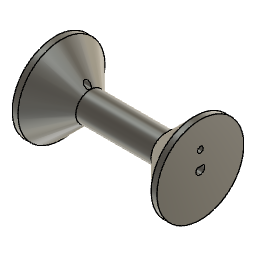
rouleau v1 (Autodesk Fusion 360 design; units mm, degrees)
Autodesk Fusion 360 part; units mm, degrees
sketch "Esquisse1" plane through (0, 0, 0) normal (0, 1, 0) x (1, 0, 0)
  line L0 (-25, -1.5) -> (-25, -15)
  line L1 (-25, -15) -> (-23, -15)
  line L2 (-23, -15) -> (-13.0387, -5)
  line L3 (-13.0387, -5) -> (12.9612, -5)
  line L4 (12.9612, -5) -> (23, -15)
  line L5 (23, -15) -> (25, -15)
  line L6 (25, -15) -> (25, -1.5)
  line L7 (25, -1.5) -> (-25, -1.5)
  constraint vertical L0
  constraint perpendicular L0 L1
  constraint perpendicular L0 L3
  constraint perpendicular L2 L4
  constraint parallel L1 L5
  constraint perpendicular L5 L6
  constraint coincident L0 L7.end
  constraint perpendicular L0 L7
revolve "Révolution1" add sketch "Esquisse1" angle 360 about axis through (1.75, 0, 0) along (1, 0, 0)
sketch "Esquisse2" plane through (-25, 0, 0) normal (-1, 0, 0) x (0, -1, 0)
  circle A0 centre (0, 0) radius 15
  circle A1 centre (0, 0) radius 1.5
  line L0 (1.1208, 0.9969) -> (-1.1208, 0.9969)
  arc A2 (1.1208, 0.9969) -> (-1.1208, 0.9969) centre (0, 0) ccw
  constraint coincident A1 L0.start
  constraint coincident A1 L0.end
  constraint horizontal L0
  constraint coincident A0.centre A1.centre
extrude "Extrusion1" add sketch "Esquisse2" against normal up to surface (50 mm away) contours A1 L0 A2
sketch "Esquisse3" plane through (-25, 0, 0) normal (-1, 0, 0) x (0, -1, 0)
  circle A0 centre (0, 0) radius 15
  arc A1 (-1.1208, 0.9969) -> (1.1208, 0.9969) centre (0, 0) ccw
  line L0 (-1.1208, 0.9969) -> (1.1208, 0.9969)
  circle A2 centre (0, 6) radius 0.9805
extrude "Extrusion2" cut sketch "Esquisse3" against normal up to surface (50 mm away) contours A2
